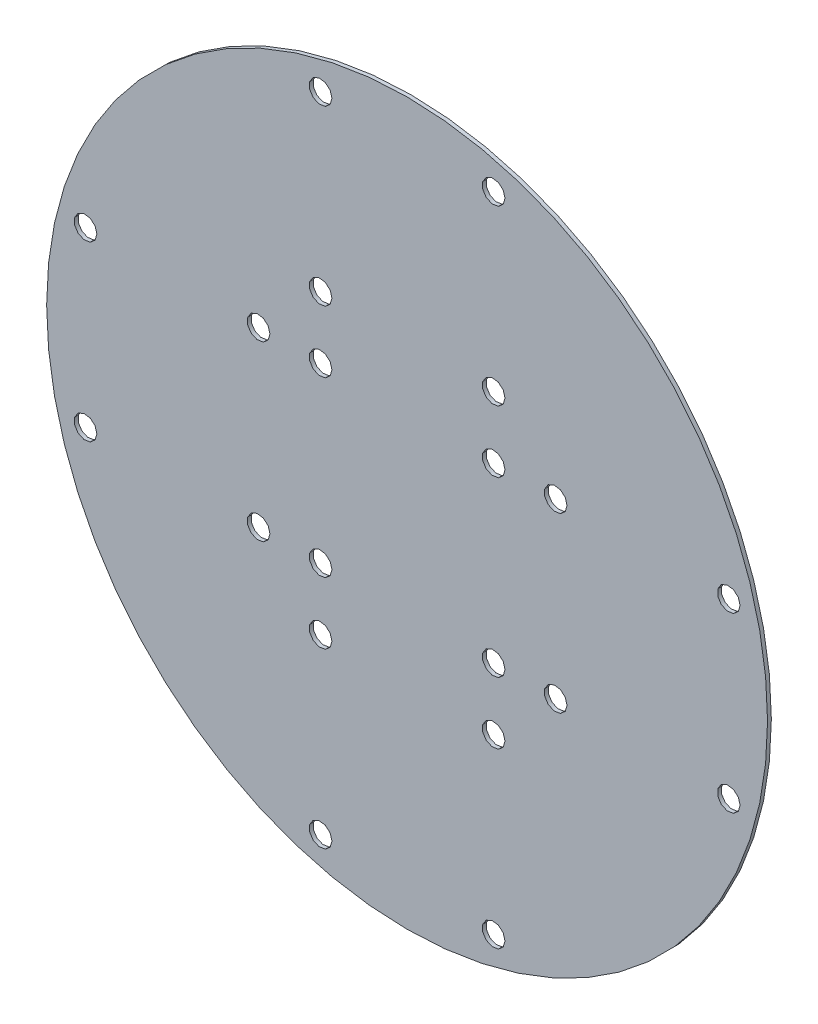
# Autodesk Inventor part: Net_Filter
Saved by Autodesk Inventor 2020 (Build 240168000, 168)
## iProperties
Created: 2021-06-02
Part Number: Net_Filter
Material: Generic
Document SubType Name: Modeling
Designer: Workshop
Density: 1 g/cm^3
Appearance: PTFE
Author: Workshop
Autodesk Inventor part; units mm, degrees
ref_plane "YZ Plane" through (0, 0, 0) normal (1, 0, 0) x (0, 1, 0)
ref_plane "XZ Plane" through (0, 0, 0) normal (0, 1, 0) x (-1, 0, 0)
ref_plane "XY Plane" through (0, 0, 0) normal (0, 0, 1) x (1, 0, 0)
sketch "Sketch1" plane through (0, 0, 0) normal (0, 0, 1) x (1, 0, 0)
  circle A0 centre (42.378, -11.4019) radius 1.5 projected
  circle A1 centre (42.3781, 11.4023) radius 1.5 projected
  circle A2 centre (-11.4017, -42.3778) radius 1.5 projected
  circle A3 centre (11.4025, -42.3779) radius 1.5 projected
  circle A4 centre (-42.3776, 11.4019) radius 1.5 projected
  circle A5 centre (-42.3777, -11.4022) radius 1.5 projected
  circle A6 centre (11.4021, 42.3779) radius 1.5 projected
  circle A7 centre (0, 0) radius 47.5 projected
  circle A8 centre (-11.4021, 42.3779) radius 1.5 projected
  circle A9 centre (19.5737, -11.4021) radius 1.5 projected
  circle A10 centre (19.5736, 11.4021) radius 1.5 projected
  circle A11 centre (-11.4021, -19.5737) radius 1.5 projected
  circle A12 centre (11.4021, -19.5736) radius 1.5 projected
  circle A13 centre (-19.5737, 11.4021) radius 1.5 projected
  circle A14 centre (-19.5736, -11.4021) radius 1.5 projected
  circle A15 centre (11.4021, 19.5737) radius 1.5 projected
  circle A16 centre (-11.4021, 19.5736) radius 1.5 projected
  circle A17 centre (11.4021, 11.4021) radius 1.5 projected
  circle A18 centre (11.4021, -11.4021) radius 1.5 projected
  circle A19 centre (-11.4021, -11.4021) radius 1.5 projected
  circle A20 centre (-11.4021, 11.4021) radius 1.5 projected
extrude "Extrusion1" add sketch "Sketch1" along normal mid plane 0.5
body "Solid1"
